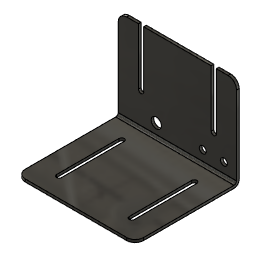
K51 Collective Module (Autodesk Fusion 360 archive; units mm, degrees)
design "K-51 Mounting Bracket"
Autodesk Fusion 360 part; units mm, degrees
sketch "Sketch1" plane through (0, 0, 0) normal (0, 1, 0) x (1, 0, 0)
  line L0 (0, 0) -> (140, 0)
  line L1 (140, 0) -> (140, -120)
  line L2 (140, -120) -> (0, -120)
  line L3 (0, -120) -> (0, 0)
  line L4 (70, 0) -> (70, -120) construction
  line L5 (23.95, -23) -> (30.05, -23) construction
  line L6 (30.05, -23) -> (30.05, -60)
  line L7 (23.95, -60) -> (23.95, -23)
  line L8 (0, -60) -> (140, -60) construction
  arc A0 (30.05, -23) -> (23.95, -23) centre (27, -23) ccw
  arc A1 (23.95, -97) -> (30.05, -97) centre (27, -97) ccw
  line L9 (23.95, -60) -> (23.95, -97)
  line L10 (30.05, -97) -> (30.05, -60)
  arc A2 (116.05, -23) -> (109.95, -23) centre (113, -23) ccw
  line L11 (116.05, -60) -> (116.05, -23)
  line L12 (109.95, -23) -> (109.95, -60)
  line L13 (116.05, -60) -> (116.05, -97)
  line L14 (109.95, -97) -> (109.95, -60)
  arc A3 (109.95, -97) -> (116.05, -97) centre (113, -97) ccw
  point P0 (27, -23)
  dimension "d1" = 140
  dimension "d2" = 120
  dimension "d3" = 37
  dimension "d4" = 6.1
  dimension "d5" = 43
  constraint horizontal L0
  constraint vertical L1
  constraint horizontal L2
  constraint vertical L3
  constraint coincident L0.start L3.end
  constraint midpoint L0 L4.start
  constraint midpoint L2 L4.end
  constraint horizontal L5
  constraint vertical L6
  constraint vertical L7
  constraint midpoint L3 L8.start
  constraint midpoint L1 L8.end
  constraint coincident L6.end L8
  constraint coincident L7.start L8
  constraint midpoint L5 P0
  constraint coincident P0 A0.centre
  constraint symmetric L5.start L8 A1.start
  constraint symmetric L5.end L8 A1.end
  constraint symmetric L6.end L8 L10.end
  constraint symmetric L7.start L8 L9.start
  constraint symmetric L8 A0 A1
  constraint symmetric L4 L5.start A2.start
  constraint symmetric L4 L5.end A2.end
  constraint symmetric L4 L6.end L12.end
  constraint symmetric L4 L7.start L11.start
  constraint symmetric L4 A0 A2
  constraint symmetric L4 A1.end L14.start
  constraint symmetric L4 A1.start L13.end
  constraint symmetric L4 A1 A3
  measures "d1" distance of L0.start L0.end
  measures "d2" distance of L0.start L2.end
  measures "d3" distance of L5.start L7.start
  measures "d4" distance of L5.start L5.end
  measures "d5" distance of L4 P0
surface "SurfacePatch1" add patch profiles "Sketch1" section 1 makes body 1
sketch "Sketch2" plane through (0, 0, 0) normal (0, 0, 1) x (1, 0, 0)
  line L0 (140, 0) -> (0, 0)
  line L1 (0, 0) -> (0, 106)
  line L2 (0, 106) -> (140, 106) construction
  line L3 (140, 106) -> (140, 0)
  line L4 (70, 106) -> (70, 0) construction
  line L5 (23.95, 106) -> (23.95, 39)
  line L6 (30.05, 106) -> (30.05, 39)
  line L7 (30.05, 39) -> (23.95, 39) construction
  arc A0 (23.95, 39) -> (30.05, 39) centre (27, 39) ccw
  line L8 (0, 106) -> (23.95, 106)
  line L9 (30.05, 106) -> (70, 106)
  line L10 (140, 106) -> (116.05, 106)
  line L11 (116.05, 106) -> (116.05, 39)
  arc A1 (109.95, 39) -> (116.05, 39) centre (113, 39) ccw
  line L12 (109.95, 106) -> (109.95, 39)
  line L13 (109.95, 106) -> (70, 106)
  dimension "d6" = 106
  dimension "d7" = 6.1
  dimension "d8" = 43
  dimension "d9" = 67
  constraint coincident L0.end L1.start
  constraint perpendicular L0 L1
  constraint perpendicular L1 L2
  constraint coincident L0.start L3.end
  constraint vertical L3
  constraint midpoint L2 L4.start
  constraint midpoint L0 L4.end
  constraint coincident L2 L5.start
  constraint perpendicular L2 L5
  constraint coincident L2 L6.start
  constraint perpendicular L2 L6
  constraint horizontal L7
  constraint midpoint L7 A0.centre
  constraint symmetric L1.end L4 L2.end
  constraint symmetric L9.end L4 L13.end
  constraint symmetric L4 L5.start L10.end
  constraint symmetric L4 L5.end L11.end
  constraint symmetric L4 L6.start L12.start
  constraint symmetric L4 L6.end A1.start
  constraint symmetric L4 A0 A1
  measures "d6" distance of L2.end L0.start
  measures "d7" distance of L5.end L6.end
  measures "d8" distance of L4 A0.centre
  measures "d9" distance of L2 A0.centre
surface "SurfacePatch2" add patch profiles "Sketch2" section 1 separate body makes body 2
stitch "SurfaceStitch1" surfaces 1 2 tolerance 0.1 makes body 3
fillet "Fillet1" radius 3 1 edges at (70, 0, 0) on bodies 3
thicken "Thicken1" add thickness -3.1 3 faces at (70, 61.3333, 0) (46.6667, 2.8573, 0.0034) (83.3167, 0, 35.3333) separate body on bodies 3 makes body 4
fillet "Fillet2" radius 10 4 edges at (140, -1.55, 120) (140, 106, -1.55) (0, 106, -1.55) (0, -1.55, 120) on bodies 4
sketch "Sketch3" plane through (0, 0, 0) normal (0, 0, 1) x (1, 0, 0)
  circle A0 centre (125, 14.9) radius 4.1
  line L0 (130, -3.1) -> (10, -3.1)
  line L1 (140, 96) -> (140, 3)
  circle A1 centre (100, 14.9) radius 4.1
  circle A2 centre (45, 14.9) radius 6.1
  circle A3 centre (5, 14.9) radius 6.1
  dimension "d16" = 18
  dimension "d17" = 15
  dimension "d18" = 8.2
  dimension "d19" = 25
  dimension "d21" = 12.2
  dimension "d22" = 55
  dimension "d23" = 40
  constraint horizontal A0.centre A1.centre
  constraint equal A0 A1
  constraint horizontal A1.centre A2.centre
  constraint horizontal A2.centre A3.centre
  constraint equal A2 A3
  measures "d16" distance of A0.centre L0
  measures "d17" distance of A0.centre L1
  measures "d18" diameter of A0
  measures "d19" distance of A0.centre A1.centre
  measures "d21" diameter of A2
  measures "d22" horizontal distance of A1.centre A2.centre
  measures "d23" horizontal distance of A2.centre A3.centre
extrude "Extrude1" cut sketch "Sketch3" against normal through all contours A0 | A1 | A2 bodies 4
hidden bodies 3
equation "d3 = ( 74 / 2 ) * 1 mm"
equation "d5 = ( 86 / 2 ) * 1 mm"
equation "d8 = ( 86 / 2 ) * 1 mm"

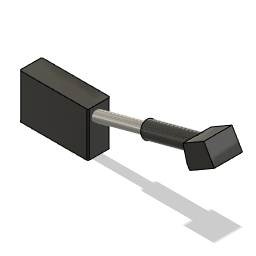
design "K-51 Collective"
Autodesk Fusion 360 part; units mm, degrees
ref_plane "WorkPlane1" through (0, 0, 21.7) normal (0, 0, 1) x (1, 0, 0)
sketch "Sketch1" plane through (0, 0, 21.7) normal (0, 0, 1) x (1, 0, 0)
  line L0 (48, 36) -> (-122, 36)
  line L1 (-122, 36) -> (-122, -74)
  line L2 (-122, -74) -> (48, -74)
  line L3 (48, -74) -> (48, 36)
  dimension "d1" = 170
  dimension "d2" = 110
  dimension "d3" = 48
  dimension "d4" = 36
  constraint horizontal L0
  constraint vertical L1
  constraint horizontal L2
  constraint vertical L3
  measures "d1" distance of L0.start L0.end
  measures "d2" distance of L0.start L2.end
  measures "d3" distance of origin L3
  measures "d4" distance of origin L0
extrude "Extrude1" add sketch "Sketch1" against normal blind 55 makes body 1
sketch "Sketch2" plane through (0, 0, 0) normal (0, 0, 1) x (1, 0, 0)
  line L0 (0, 0) -> (309.0963, 82.8221) construction
  line L1 (309.0963, 82.8221) -> (314.2726, 63.5036)
  line L2 (314.2726, 63.5036) -> (320.9541, 51.9309)
  line L3 (320.9541, 51.9309) -> (381.8814, 87.1073)
  line L4 (381.8814, 87.1073) -> (355.8814, 132.1406)
  line L5 (355.8814, 132.1406) -> (303.9199, 102.1406)
  line L6 (303.9199, 102.1406) -> (309.0963, 82.8221)
  line L7 (1.75, 0) -> (22.5, 0)
  point P0 (-122, 36)
  dimension "d8" = 320
  dimension "d9" = 20
  dimension "d10" = 20
  dimension "d11" = 60
  dimension "d12" = 52
  dimension "d13" = 15
  dimension "d14" = 15
  dimension "d25" = 503.8814
  constraint coincident L0.start origin
  constraint perpendicular L0 L1
  constraint perpendicular L2 L3
  constraint perpendicular L3 L4
  constraint perpendicular L2 L5
  constraint perpendicular L0 L6
  measures "d8" distance of L0.start L0.end
  measures "d9" distance of L0.end L1.end
  measures "d10" distance of L0.end L5.end
  measures "d11" distance of L4.end L5.end
  measures "d12" distance of L3.end L4.end
  measures "d13" angle of L0 L7
  measures "d14" angle of L0 L5
  measures "d25" horizontal distance of L3.end P0
extrude "Extrude2" add sketch "Sketch2" against normal blind 28 separate body makes body 2
move_face "OffsetFaces1" offset 42 1 faces at (348.953, 100.69, 0) on bodies 2
sketch "Sketch3" plane through (309.0963, 82.8221, 0) normal (-0.965926, -0.258819, 0) x (0, 0, 1)
  line L0 (42, -20) -> (42, 20)
  line L1 (42, 20) -> (-28, 20)
  line L2 (-28, 20) -> (-28, -20)
  line L3 (-28, -20) -> (42, -20)
  circle A0 centre (0, 0) radius 20
  dimension "d18" = 40
  constraint coincident A0.centre origin
  measures "d18" diameter of A0
extrude "Extrude3" add sketch "Sketch3" along normal blind 136 separate body contours A0 makes body 3
sketch "Sketch4" plane through (177.7304, 47.6227, 0) normal (-0.965926, -0.258819, 0) x (0, 0, 1)
  circle A0 centre (0, 0) radius 20
  circle A1 centre (0, 0) radius 12.7
  dimension "d22" = 25.4
  constraint coincident A0.centre A1.centre
  measures "d22" diameter of A1
extrude "Extrude4" add sketch "Sketch4" along normal up to surface (184 mm away) separate body contours A1 makes body 4
fillet "Fillet1" radius 3 4 edges at (48, -19, 21.7) (48, -19, -33.3) (-122, -19, -33.3) (-122, -19, 21.7) on bodies 1
equation "d5 = ( 25.4 / 2 ) * 1 mm + 9 mm"
equation "d17 = 70 mm - 28 mm"
